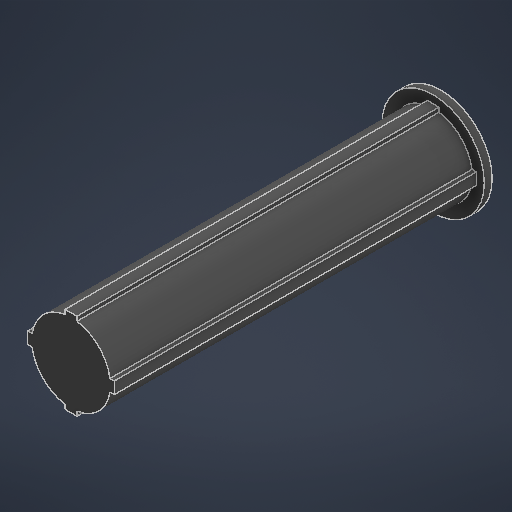
# Autodesk Inventor part: HIN-61 BISAGRA (BUJE PLASTICO)
Saved by Autodesk Inventor 2025 (Build 290162000, 162)
## iProperties
Created: 2026-02-11
Part Number: HIN-61 BISAGRA (BUJE PLASTICO)
Material: Plástico ABS
Document SubType Name: Modeling
Designer: ROLANDO
Density: 1.06 g/cm^3
Appearance: Genérico
Author: ROLANDO
Autodesk Inventor part; units mm, degrees
ref_plane "YZ Plane" through (0, 0, 0) normal (1, 0, 0) x (0, 1, 0)
ref_plane "XZ Plane" through (0, 0, 0) normal (0, 1, 0) x (-1, 0, 0)
ref_plane "XY Plane" through (0, 0, 0) normal (0, 0, 1) x (1, 0, 0)
sketch "Boceto1" plane through (0, 0, 0) normal (0, 0, 1) x (1, 0, 0)
  line L0 (0, 12.1119) -> (0, -11.4197) construction
  line L1 (-11.1817, 0) -> (11.1817, 0) construction
  line L2 (4.9434, 0.75) -> (5.5, 0.75)
  line L3 (4.9434, -0.75) -> (5.5, -0.75)
  line L4 (5.5, -0.75) -> (5.5, 0.75)
  line L5 (-0.75, 4.9434) -> (-0.75, 5.5)
  line L6 (0.75, 5.5) -> (-0.75, 5.5)
  line L7 (0.75, 4.9434) -> (0.75, 5.5)
  line L8 (-4.9434, -0.75) -> (-5.5, -0.75)
  line L9 (-5.5, 0.75) -> (-5.5, -0.75)
  line L10 (-4.9434, 0.75) -> (-5.5, 0.75)
  line L11 (0.75, -4.9434) -> (0.75, -5.5)
  line L12 (-0.75, -5.5) -> (0.75, -5.5)
  line L13 (-0.75, -4.9434) -> (-0.75, -5.5)
  arc A0 (-0.75, 4.9434) -> (-4.9434, 0.75) centre (0, 0) ccw
  arc A1 (-4.9434, -0.75) -> (-0.75, -4.9434) centre (0, 0) ccw
  arc A2 (0.75, -4.9434) -> (4.9434, -0.75) centre (0, 0) ccw
  arc A3 (4.9434, 0.75) -> (0.75, 4.9434) centre (0, 0) ccw
  circle A4 centre (0, 0) radius 5 construction
  point P0 (5.5, 0)
  dimension "d3" = 0.75
  dimension "d4" = 1.5
  dimension "d5" = 360
  dimension "d7" = 0.5
  dimension "d8" = 5
  dimension "d43" = 10
  constraints: 28 end point, 8 point on circle, 5 centre point, 4 midpoint, 3 horizontal, 2 coincident, 2 point on line, 2 vertical, 1 perpendicular, 29 other
  measures "d3" distance between parallel lines of L1 L3
  measures "d4" distance between parallel lines of L3 L2
  measures "d7" distance edge to line of A4 L6
  measures "d8" radius of A3
  measures "d43" diameter of A4
extrude "Extrusión1" add sketch "Boceto1" against normal blind 46
sketch "Boceto3" plane through (0, 0, -46) normal (0, 0, -1) x (-1, 0, 0)
  circle A0 centre (0, 0) radius 6.5
  dimension "d49" = 13
  constraints: 1 centre point, 1 coincident
  measures "d49" diameter of A0
extrude "Extrusión3" add sketch "Boceto3" along normal blind 1
sketch "Boceto2" plane through (0, 0, -47) normal (0, 0, -1) x (-1, 0, 0)
  circle A0 centre (0, 0) radius 3.5
  dimension "d46" = 7
  constraints: 1 centre point, 1 coincident
  measures "d46" diameter of A0
extrude "Extrusión2" cut sketch "Boceto2" against normal blind 40
